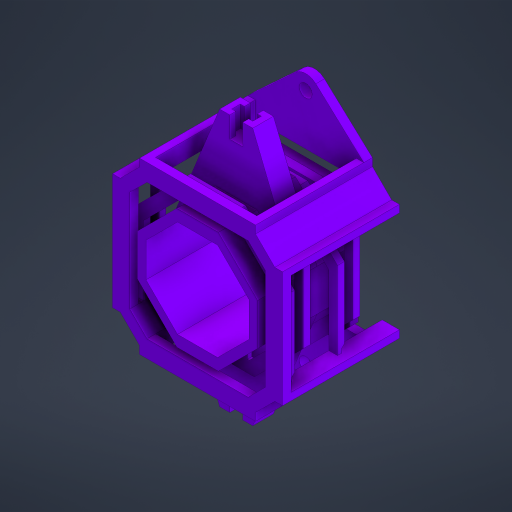
# Autodesk Inventor part: Z Axis Sample V1
Saved by Autodesk Inventor 2023.4 (Build 274418000, 418)
## iProperties
Created: 2022-08-08
Part Number: Z Axis Sample V1
Material: Generic
Document SubType Name: Modeling
Designer: xSibe
Density: 1 g/cm^3
Appearance: Plastic Purple
Author: xSibe
Autodesk Inventor part; units mm, degrees
ref_plane "YZ Plane" through (0, 0, 0) normal (1, 0, 0) x (0, 1, 0)
ref_plane "XZ Plane" through (0, 0, 0) normal (0, 1, 0) x (-1, 0, 0)
ref_plane "XY Plane" through (0, 0, 0) normal (0, 0, 1) x (1, 0, 0)
sketch "Sketch1" plane through (0, 0, 0) normal (0, 0, 1) x (1, 0, 0)
  circle A0 centre (-10, 20.9) radius 1.875 projected
  circle A1 centre (-10, -20.9) radius 1.875 projected
  circle A2 centre (10, 20.9) radius 1.875 projected
  circle A3 centre (10, -20.9) radius 1.875 projected
  circle A4 centre (20.8, -14.4) radius 2.075 projected
  circle A5 centre (20.8, 14.4) radius 2.075 projected
  circle A6 centre (-20.8, 14.4) radius 2.075 projected
  circle A7 centre (-20.8, -14.4) radius 2.075 projected
  line L0 (16.9, -16.9) -> (-16.9, -16.9) projected
  line L1 (-16.9, -16.9) -> (-16.9, 16.9) projected
  line L2 (-16.9, 16.9) -> (16.9, 16.9) projected
  line L3 (16.9, 16.9) -> (16.9, -16.9) projected
  line L4 (-17.05, 24.9) -> (-17.05, 22.55) projected
  line L5 (-17.05, 22.55) -> (-22.55, 17.05) projected
  line L6 (-22.55, 17.05) -> (-24.9, 17.05) projected
  line L7 (-24.9, 17.05) -> (-24.9, -17.05) projected
  line L8 (-24.9, -17.05) -> (-22.55, -17.05) projected
  line L9 (-22.55, -17.05) -> (-17.05, -22.55) projected
  line L10 (-17.05, -22.55) -> (-17.05, -24.9) projected
  line L11 (-17.05, -24.9) -> (17.05, -24.9) projected
  line L12 (17.05, -24.9) -> (17.05, -22.55) projected
  line L13 (17.05, -22.55) -> (22.55, -17.05) projected
  line L14 (22.55, -17.05) -> (24.9, -17.05) projected
  line L15 (24.9, -17.05) -> (24.9, 17.05) projected
  line L16 (24.9, 17.05) -> (22.55, 17.05) projected
  line L17 (22.55, 17.05) -> (17.05, 22.55) projected
  line L18 (17.05, 22.55) -> (17.05, 24.9) projected
  line L19 (17.05, 24.9) -> (-17.05, 24.9) projected
  line L20 (24.725, 16.875) -> (24.725, -16.875)
  line L21 (24.725, -16.875) -> (22.4775, -16.875)
  line L22 (22.4775, -16.875) -> (16.875, -22.4775)
  line L23 (16.875, -22.4775) -> (16.875, -24.725)
  line L24 (16.875, -24.725) -> (-16.875, -24.725)
  line L25 (-16.875, -24.725) -> (-16.875, -22.4775)
  line L26 (-16.875, -22.4775) -> (-22.4775, -16.875)
  line L27 (-22.4775, -16.875) -> (-24.725, -16.875)
  line L28 (-24.725, -16.875) -> (-24.725, 16.875)
  line L29 (-24.725, 16.875) -> (-22.4775, 16.875)
  line L30 (-22.4775, 16.875) -> (-16.875, 22.4775)
  line L31 (-16.875, 22.4775) -> (-16.875, 24.725)
  line L32 (-16.875, 24.725) -> (16.875, 24.725)
  line L33 (16.875, 24.725) -> (16.875, 22.4775)
  line L34 (16.875, 22.4775) -> (22.4775, 16.875)
  line L35 (22.4775, 16.875) -> (24.725, 16.875)
  circle A8 centre (0, 0) radius 12.5
  line L36 (24.725, -16.875) -> (24.725, -24.725)
  line L37 (24.725, -24.725) -> (16.875, -24.725)
  line L38 (24.725, -24.725) -> (14.725, -24.725)
  line L39 (14.725, -24.725) -> (14.725, -19.725)
  line L40 (19.725, -14.725) -> (24.725, -14.725)
  line L41 (24.725, -14.725) -> (24.725, -24.725)
  line L42 (19.725, -14.725) -> (14.725, -19.725)
  line L43 (24.725, 14.725) -> (19.725, 14.725)
  line L44 (14.725, 19.725) -> (19.725, 14.725)
  line L45 (14.725, 19.725) -> (14.725, 24.725)
  line L46 (14.725, 24.725) -> (24.725, 24.725)
  line L47 (24.725, 24.725) -> (24.725, 14.725)
  line L48 (-14.725, 24.725) -> (-14.725, 19.725)
  line L49 (-19.725, 14.725) -> (-14.725, 19.725)
  line L50 (-19.725, 14.725) -> (-24.725, 14.725)
  line L51 (-24.725, 14.725) -> (-24.725, 24.725)
  line L52 (-24.725, 24.725) -> (-14.725, 24.725)
  line L53 (-24.725, -14.725) -> (-19.725, -14.725)
  line L54 (-14.725, -19.725) -> (-19.725, -14.725)
  line L55 (-14.725, -19.725) -> (-14.725, -24.725)
  line L56 (-14.725, -24.725) -> (-24.725, -24.725)
  line L57 (-24.725, -24.725) -> (-24.725, -14.725)
  line L58 (14.725, -19.725) -> (-14.725, -19.725)
  line L59 (-14.725, -19.725) -> (-14.725, -24.725)
  line L60 (-14.725, -24.725) -> (14.725, -24.725)
  line L61 (14.725, -24.725) -> (14.725, -19.725)
  line L62 (-19.725, -14.725) -> (-24.725, -14.725)
  line L63 (-24.725, -14.725) -> (-24.725, 14.725)
  line L64 (-24.725, 14.725) -> (-19.725, 14.725)
  line L65 (-19.725, 14.725) -> (-19.725, -14.725)
  line L66 (-14.725, 19.725) -> (14.725, 19.725)
  line L67 (14.725, 19.725) -> (14.725, 24.725)
  line L68 (14.725, 24.725) -> (-14.725, 24.725)
  line L69 (-14.725, 24.725) -> (-14.725, 19.725)
  line L70 (19.725, 14.725) -> (24.725, 14.725)
  line L71 (24.725, 14.725) -> (24.725, -14.725)
  line L72 (24.725, -14.725) -> (19.725, -14.725)
  line L73 (19.725, -14.725) -> (19.725, 14.725)
  point P0 (16.875, -16.875)
  point P1 (14.725, -14.725)
  dimension "d0" = 0.175
  dimension "d3" = 25
  dimension "d24" = 10
  dimension "d25" = 10
  dimension "d26" = 5
  dimension "d27" = 5
  dimension "d30" = 360
  constraints: 108 end point, 10 parallel, 6 perpendicular, 5 horizontal, 2 point on line, 1 centre point, 1 coincident, 1 vertical, 56 other
  measures "d0" distance between parallel lines of L15 L20
  measures "d3" diameter of A8
  measures "d24" distance of point (14.725, -14.725) L40.end
  measures "d25" distance of L38.end point (14.725, -14.725)
  measures "d26" distance of L40.start point (14.725, -14.725)
  measures "d27" distance of L39.end point (14.725, -14.725)
ref_plane "Work Plane1" through (-24.9, -24.9, 7.7) normal (0, 0, 1) x (1, 0, 0)
extrude "Extrusion1" add sketch "Sketch1" along normal blind 2.5 from surface at 7.7 contours A0 L66 | A0 L66 L48 L32 L45 A2 | L49 A6 L50 L28 L29 L30 L31 L32 L48 | A2 L66 | L49 L50 A6 | L32 L33 L34 L35 L20 L43 A5 L44 L45 | L50 L65 A6 | A6 L65 A7 L53 L28 L50 | A5 L43 L44 | L65 L53 A7 | L53 A7 L54 L55 L24 L25 L26 L27 L28 | L43 L20 L40 A4 L73 A5 | A5 L73 L43 | L53 L54 A7 | A4 L40 L73 | L20 L21 L22 L23 L24 L39 L42 A4 L40 | L42 L40 A4 | L58 A1 A3 L39 L24 L55 | L58 A1 | A3 L58 picked at (-10.1758, 21.5261) picked at (10.0076, 20.8619) picked at (-9.9136, -20.7357) picked at (10.3659, -21.7168)
sketch "Sketch2" plane through (0, 0, 0) normal (0, 0, 1) x (1, 0, 0)
  line L0 (22.4775, 16.875) -> (24.725, 16.875) projected
  line L1 (16.875, 22.4775) -> (22.4775, 16.875) projected
  line L2 (16.875, 24.725) -> (16.875, 22.4775) projected
  line L3 (-16.875, 24.725) -> (16.875, 24.725) projected
  line L4 (-16.875, 22.4775) -> (-16.875, 24.725) projected
  line L5 (-22.4775, 16.875) -> (-16.875, 22.4775) projected
  line L6 (-24.725, 16.875) -> (-22.4775, 16.875) projected
  line L7 (-24.725, -16.875) -> (-24.725, 16.875) projected
  line L8 (-22.4775, -16.875) -> (-24.725, -16.875) projected
  line L9 (-16.875, -22.4775) -> (-22.4775, -16.875) projected
  line L10 (-16.875, -24.725) -> (-16.875, -22.4775) projected
  line L11 (16.875, -24.725) -> (-16.875, -24.725) projected
  line L12 (16.875, -22.4775) -> (16.875, -24.725) projected
  line L13 (22.4775, -16.875) -> (16.875, -22.4775) projected
  line L14 (24.725, -16.875) -> (22.4775, -16.875) projected
  line L15 (24.725, 16.875) -> (24.725, -16.875) projected
  line L16 (-16.875, -24.725) -> (-24.725, -24.725)
  line L17 (-24.725, -24.725) -> (-24.725, -16.875)
  line L18 (-24.725, -24.725) -> (-14.725, -24.725)
  line L19 (-14.725, -24.725) -> (-14.725, -19.725)
  line L20 (-19.725, -14.725) -> (-24.725, -14.725)
  line L21 (-24.725, -14.725) -> (-24.725, -24.725)
  line L22 (-14.725, -19.725) -> (-19.725, -14.725)
  line L23 (24.725, -14.725) -> (19.725, -14.725)
  line L24 (19.725, -14.725) -> (14.725, -19.725)
  line L25 (14.725, -19.725) -> (14.725, -24.725)
  line L26 (24.725, -24.725) -> (16.875, -24.725)
  line L27 (24.725, -24.725) -> (24.725, -14.725)
  line L28 (14.725, 24.725) -> (14.725, 19.725)
  line L29 (14.725, 19.725) -> (19.725, 14.725)
  line L30 (19.725, 14.725) -> (24.725, 14.725)
  line L31 (24.725, 24.725) -> (24.725, 16.875)
  line L32 (24.725, 24.725) -> (14.725, 24.725)
  line L33 (-24.725, 14.725) -> (-19.725, 14.725)
  line L34 (-19.725, 14.725) -> (-14.725, 19.725)
  line L35 (-14.725, 19.725) -> (-14.725, 24.725)
  line L36 (-24.725, 24.725) -> (-16.875, 24.725)
  line L37 (-24.725, 24.725) -> (-24.725, 14.725)
  line L38 (24.725, 14.725) -> (19.725, 14.725)
  line L39 (19.725, 14.725) -> (19.725, -14.725)
  line L40 (19.725, -14.725) -> (24.725, -14.725)
  line L41 (24.725, -14.725) -> (24.725, 14.725)
  line L42 (14.725, -19.725) -> (-14.725, -19.725)
  line L43 (-14.725, -19.725) -> (-14.725, -24.725)
  line L44 (-14.725, -24.725) -> (14.725, -24.725)
  line L45 (14.725, -24.725) -> (14.725, -19.725)
  line L46 (-19.725, -14.725) -> (-24.725, -14.725)
  line L47 (-24.725, -14.725) -> (-24.725, 14.725)
  line L48 (-24.725, 14.725) -> (-19.725, 14.725)
  line L49 (-19.725, 14.725) -> (-19.725, -14.725)
  line L50 (-14.725, 19.725) -> (14.725, 19.725)
  line L51 (14.725, 19.725) -> (14.725, 24.725)
  line L52 (14.725, 24.725) -> (-14.725, 24.725)
  line L53 (-14.725, 24.725) -> (-14.725, 19.725)
  point P0 (0, 0)
  point P1 (-14.725, -14.725)
  dimension "d12" = 10
  dimension "d13" = 10
  dimension "d14" = 5
  dimension "d15" = 5
  dimension "d18" = 360
  constraints: 76 end point, 10 parallel, 6 horizontal, 6 perpendicular, 2 point on line, 45 other
  measures "d12" distance of L20.end point (-14.725, -14.725)
  measures "d13" distance of point (-14.725, -14.725) L18.end
  measures "d14" distance of L19.end point (-14.725, -14.725)
  measures "d15" distance of L20.start point (-14.725, -14.725)
extrude "Extrusion2" add sketch "Sketch2" along normal blind 31.5 from surface at 10.2 contours L0 L15 L30 L29 L28 L3 L2 L1 | L15 L14 L13 L12 L11 L25 L24 L23 | L35 L34 L33 L7 L6 L5 L4 L3 | L19 L11 L10 L9 L8 L7 L20 L22
extrude "Extrusion3" add sketch "Sketch2" against normal blind 2.5 from surface at 41.7 contours L15 L23 L39 L30 | L28 L50 L35 L3 | L25 L11 L19 L42 | L49 L20 L7 L33
sketch "Sketch3" plane through (0, 0, 0) normal (0, 0, 1) x (1, 0, 0)
  line L0 (-14.725, 19.725) -> (-19.725, 14.725) projected
  line L1 (14.725, 19.725) -> (-14.725, 19.725) projected
  line L2 (19.725, 14.725) -> (14.725, 19.725) projected
  line L3 (14.725, -19.725) -> (19.725, -14.725) projected
  line L4 (-14.725, -19.725) -> (14.725, -19.725) projected
  line L5 (-19.725, -14.725) -> (-14.725, -19.725) projected
  line L6 (-24.725, -16.875) -> (-24.725, 16.875) projected
  line L7 (-22.4775, -16.875) -> (-24.725, -16.875) projected
  line L8 (-16.875, -22.4775) -> (-22.4775, -16.875) projected
  line L9 (-16.875, -24.725) -> (-16.875, -22.4775) projected
  line L10 (16.875, -24.725) -> (-16.875, -24.725) projected
  line L11 (16.875, -22.4775) -> (16.875, -24.725) projected
  line L12 (22.4775, -16.875) -> (16.875, -22.4775) projected
  line L13 (24.725, -16.875) -> (22.4775, -16.875) projected
  line L14 (24.725, 16.875) -> (24.725, -16.875) projected
  line L15 (22.4775, 16.875) -> (24.725, 16.875) projected
  line L16 (16.875, 22.4775) -> (22.4775, 16.875) projected
  line L17 (16.875, 24.725) -> (16.875, 22.4775) projected
  line L18 (-16.875, 24.725) -> (16.875, 24.725) projected
  line L19 (-16.875, 22.4775) -> (-16.875, 24.725) projected
  line L20 (-22.4775, 16.875) -> (-16.875, 22.4775) projected
  line L21 (-24.725, 16.875) -> (-22.4775, 16.875) projected
  circle A0 centre (0, 0) radius 13.25
  circle A1 centre (0, 0) radius 18.25
  line L22 (13.25, 18.25) -> (-13.25, 18.25)
  line L23 (-18.25, 13.25) -> (-18.25, -13.25)
  line L24 (-13.25, -18.25) -> (13.25, -18.25)
  line L25 (18.25, -13.25) -> (18.25, 13.25)
  line L26 (18.25, 18.25) -> (-18.25, -18.25) construction
  line L27 (-18.25, 18.25) -> (18.25, -18.25) construction
  line L28 (-14.725, -19.725) -> (-14.725, -24.725) projected
  line L29 (14.725, -24.725) -> (-14.725, -24.725) projected
  line L30 (14.725, -24.725) -> (14.725, -19.725) projected
  line L31 (-14.725, -19.725) -> (14.725, -19.725) projected
  line L32 (24.725, 14.725) -> (19.725, 14.725) projected
  line L33 (19.725, -14.725) -> (19.725, 14.725) projected
  line L34 (19.725, -14.725) -> (24.725, -14.725) projected
  line L35 (24.725, 14.725) -> (24.725, -14.725) projected
  line L36 (-19.725, 14.725) -> (-24.725, 14.725) projected
  line L37 (-24.725, -14.725) -> (-24.725, 14.725) projected
  line L38 (-24.725, -14.725) -> (-19.725, -14.725) projected
  line L39 (-19.725, 14.725) -> (-19.725, -14.725) projected
  line L40 (-14.725, 24.725) -> (-14.725, 19.725) projected
  line L41 (14.725, 19.725) -> (-14.725, 19.725) projected
  line L42 (14.725, 19.725) -> (14.725, 24.725) projected
  line L43 (-14.725, 24.725) -> (14.725, 24.725) projected
  line L44 (18.25, -13.25) -> (13.25, -18.25)
  line L45 (-13.25, -18.25) -> (-18.25, -13.25)
  line L46 (-18.25, 13.25) -> (-13.25, 18.25)
  line L47 (13.25, 18.25) -> (18.25, 13.25)
  line L48 (10, 14.1625) -> (-10, 14.1625)
  line L49 (-10, 14.1625) -> (-10, -14.1625)
  line L50 (-10, -14.1625) -> (10, -14.1625)
  line L51 (10, -14.1625) -> (10, 14.1625)
  line L52 (10, 14.1625) -> (-10, -14.1625) construction
  line L53 (-10, 14.1625) -> (10, -14.1625) construction
  line L54 (5, 15) -> (-5, 15)
  line L55 (-15, 5) -> (-15, -5)
  line L56 (-5, -15) -> (5, -15)
  line L57 (15, -5) -> (15, 5)
  line L58 (15, 15) -> (-15, -15) construction
  line L59 (-15, 15) -> (15, -15) construction
  line L60 (15, -5) -> (5, -15)
  line L61 (-5, -15) -> (-15, -5)
  line L62 (-15, 5) -> (-5, 15)
  line L63 (5, 15) -> (15, 5)
  line L64 (6.0355, -17.5) -> (17.5, -6.0355)
  line L65 (17.5, -6.0355) -> (17.5, 6.0355)
  line L66 (17.5, 6.0355) -> (6.0355, 17.5)
  line L67 (6.0355, 17.5) -> (-6.0355, 17.5)
  line L68 (-6.0355, 17.5) -> (-17.5, 6.0355)
  line L69 (-17.5, 6.0355) -> (-17.5, -6.0355)
  line L70 (-17.5, -6.0355) -> (-6.0355, -17.5)
  line L71 (-6.0355, -17.5) -> (6.0355, -17.5)
  line L72 (6.0355, 17.5) -> (14, 17.5)
  line L73 (-6.0355, 17.5) -> (-14, 17.5)
  line L74 (10, 15.6625) -> (-10, 15.6625)
  line L75 (-10, 15.6625) -> (-10, 12.6625)
  line L76 (-10, 12.6625) -> (10, 12.6625)
  line L77 (10, 12.6625) -> (10, 15.6625)
  line L78 (10, 15.6625) -> (-10, 12.6625) construction
  line L79 (-10, 15.6625) -> (10, 12.6625) construction
  line L80 (10, -12.6625) -> (-10, -12.6625)
  line L81 (-10, -12.6625) -> (-10, -15.6625)
  line L82 (-10, -15.6625) -> (10, -15.6625)
  line L83 (10, -15.6625) -> (10, -12.6625)
  line L84 (10, -12.6625) -> (-10, -15.6625) construction
  line L85 (-10, -12.6625) -> (10, -15.6625) construction
  circle A2 centre (0, 0) radius 12.6625
  line L86 (-19.725, 14.725) -> (-19.725, -14.725) projected
  line L87 (19.725, -14.725) -> (19.725, 14.725) projected
  point P0 (-18.25, 10)
  point P1 (-18.25, -10)
  point P2 (18.25, -10)
  point P3 (18.25, 10)
  point P4 (15, 10.3953)
  point P5 (10.3953, 15)
  point P6 (-15, 10.3953)
  point P7 (-10.3953, 15)
  point P8 (-10.3953, -15)
  point P9 (-15, -10.3953)
  point P10 (15, -10.3953)
  point P11 (10.3953, -15)
  point P12 (10, 10)
  point P13 (10, -10)
  point P14 (-10, -10)
  point P15 (-10, 10)
  point P16 (-5.8375, -14.1625)
  point P17 (-5.8375, 14.1625)
  point P18 (5.8375, 14.1625)
  point P19 (5.8375, -14.1625)
  point P20 (0, 14.1625)
  point P21 (0, -14.1625)
  point P22 (-10, 12.6625)
  point P23 (10, 12.6625)
  point P24 (10, 14.1625)
  dimension "d32" = 26.5
  dimension "d33" = 5
  dimension "d36" = 5
  dimension "d37" = 5
  dimension "d38" = 5
  dimension "d39" = 5
  dimension "d40" = 5
  dimension "d41" = 5
  dimension "d42" = 5
  dimension "d43" = 5
  dimension "d49" = 20
  dimension "d50" = 28.325
  dimension "d57" = 30
  dimension "d58" = 30
  dimension "d59" = 10
  dimension "d60" = 10
  dimension "d61" = 10
  dimension "d62" = 10
  dimension "d63" = 10
  dimension "d64" = 10
  dimension "d65" = 10
  dimension "d66" = 10
  dimension "d67" = 2.5
  dimension "d120" = 20
  dimension "d121" = 3
  dimension "d122" = 20
  dimension "d123" = 3
  constraints: 96 end point, 19 point on line, 12 midpoint, 12 parallel, 7 perpendicular, 5 horizontal, 3 centre point, 3 tangent, 2 coincident, 7 other
  measures "d32" diameter of A0
  measures "d33" radial gap between concentric circles of A0 A1
  measures "d36" distance of L25.start L27.end
  measures "d37" distance of L24.end L27.end
  measures "d38" distance of L24.start L26.end
  measures "d39" distance of L23.end L26.end
  measures "d40" distance of L23.start L27.start
  measures "d41" distance of L22.end L27.start
  measures "d42" distance of L22.start L26.start
  measures "d43" distance of L25.end L26.start
  measures "d49" distance of L50.end L49.end
  measures "d50" distance of L49.end L48.end
  measures "d57" distance of L59.end L58.end
  measures "d58" distance of L58.end L59.start
  measures "d59" distance of L57.start L59.end
  measures "d60" distance of L56.end L59.end
  measures "d61" distance of L56.start L58.end
  measures "d62" distance of L55.end L58.end
  measures "d63" distance of L55.start L59.start
  measures "d64" distance of L54.end L59.start
  measures "d65" distance of L54.start L58.start
  measures "d66" distance of L57.end L58.start
  measures "d67" distance between parallel lines of L56 L71
  measures "d120" distance of L76.end L75.end
  measures "d121" distance of L75.end L74.end
  measures "d122" distance of L82.end L81.end
  measures "d123" distance of L81.end L80.end
ref_plane "Work Plane2" through (16.875, 24.725, 14.45) normal (0, 0, -1) x (-1, 0, 0)
extrude "Extrusion4" add sketch "Sketch3" along normal mid plane 2.5 from surface at 14.45 contours A0 L51 A2 | A0 L51 L63 L57 L60 | L51 A2 L76 A0 | A0 L76 L63 L51 | L51 L60 L80 A0 | A0 L80 A2 L51 | L76 A0 | A0 L76 L62 L48 L63 | L63 L76 L51 | L51 L66 A1 L65 L64 L60 L57 L63 | L80 L60 L50 L61 A0 | A0 L80 | L51 L80 L60 | L76 A2 L49 A0 | A0 L49 L62 L76 | L63 L48 L66 L51 L76 | L80 L61 L49 A0 | A0 L49 A2 L80 | L80 L51 L64 L50 L60 | L49 A2 A0 | A0 L49 L61 L55 L62 | L76 L49 L68 L48 L62 | L62 L49 L76 | L63 L54 L62 L48 L68 L74 L66 | L48 L62 L54 L63 | L66 L48 L51 | L51 L77 A1 L66 | L80 L49 L61 | L61 L50 L70 L49 L80 | L60 L56 L61 L50 | L50 L64 L82 L70 L61 L56 L60 | L64 A1 L83 L51 | L51 L50 L64 | L62 L55 L61 L49 L70 A1 L69 L68 | L66 L74 A1 L77 L48 | L66 L65 A1 | A1 L77 L74 L66 L72 L47 L25 L65 | L50 L83 A1 L82 L64 | L64 L65 A1 L25 L44 L24 L71 L82 L83 | A1 L65 L64 | L68 L49 L48 | L48 L75 A1 L74 L68 | L68 A1 L75 L49 | L74 L68 A1 L67 L66 | L66 A1 L74 | A1 L74 L77 | A1 L65 | L70 L82 A1 L81 L50 | L50 L49 L70 | L49 L81 A1 L70 | L82 A1 L64 | L64 A1 L71 L70 L82 | L83 L82 A1 | L74 A1 L68 | L68 L69 A1 L23 L46 L73 L74 L75 | A1 L69 L68 | A1 L67 L66 | L70 A1 L82 | L70 L69 A1 | A1 L81 L82 L70 L71 L24 L45 L23 L69 | L64 L71 A1 | L75 L74 A1 | L68 L67 A1 | L69 A1 | L67 A1 | A1 L22 L47 L72 L67 | A1 L82 L81 | A1 L71 L70 | A1 L71 | L67 L73 L46 L22 A1
extrude "Extrusion5" add sketch "Sketch3" along normal up to surface (26 mm away) from surface at 15.7 contours L63 L76 L51 | L51 L66 A1 L65 L64 L60 L57 L63 | L51 L80 L60 | L63 L48 L66 L51 L76 | L80 L51 L64 L50 L60 | L76 L49 L68 L48 L62 | L62 L49 L76 | L63 L54 L62 L48 L68 L74 L66 | L48 L62 L54 L63 | L80 L49 L61 | L61 L50 L70 L49 L80 | L60 L56 L61 L50 | L50 L64 L82 L70 L61 L56 L60 | L62 L55 L61 L49 L70 A1 L69 L68 | L66 L65 A1 | A1 L65 L64 | L74 L68 A1 L67 L66 | L64 A1 L71 L70 L82 | A1 L69 L68 | A1 L67 L66 | L70 L69 A1 | L64 L71 A1 | L68 L67 A1 | A1 L71 L70
extrude "Extrusion6" add sketch "Sketch3" against normal blind 5 from surface at 13.2 contours L76 A0 | A0 L76 L62 L48 L63 | L80 L60 L50 L61 A0 | A0 L80 | L63 L48 L66 L51 L76 | L80 L51 L64 L50 L60 | L76 L49 L68 L48 L62 | L63 L54 L62 L48 L68 L74 L66 | L48 L62 L54 L63 | L66 L48 L51 | L61 L50 L70 L49 L80 | L60 L56 L61 L50 | L50 L64 L82 L70 L61 L56 L60 | L51 L50 L64 | L66 L74 A1 L77 L48 | L50 L83 A1 L82 L64 | L68 L49 L48 | L48 L75 A1 L74 L68 | A1 L74 L77 | L70 L82 A1 L81 L50 | L50 L49 L70 | L83 L82 A1 | L75 L74 A1 | A1 L82 L81
sketch "Sketch4" plane through (0, 0, 0) normal (0, 0, 1) x (1, 0, 0)
  line L0 (-14.725, 24.725) -> (-14.725, 19.725) projected
  line L1 (14.725, 19.725) -> (-14.725, 19.725) projected
  line L2 (14.725, 19.725) -> (14.725, 24.725) projected
  line L3 (-14.725, 24.725) -> (14.725, 24.725) projected
  line L4 (24.725, 14.725) -> (19.725, 14.725) projected
  line L5 (19.725, -14.725) -> (19.725, 14.725) projected
  line L6 (19.725, -14.725) -> (24.725, -14.725) projected
  line L7 (24.725, 14.725) -> (24.725, -14.725) projected
  line L8 (-14.725, -19.725) -> (-14.725, -24.725) projected
  line L9 (14.725, -24.725) -> (-14.725, -24.725) projected
  line L10 (14.725, -24.725) -> (14.725, -19.725) projected
  line L11 (-14.725, -19.725) -> (14.725, -19.725) projected
  line L12 (-19.725, 14.725) -> (-24.725, 14.725) projected
  line L13 (-24.725, -14.725) -> (-24.725, 14.725) projected
  line L14 (-24.725, -14.725) -> (-19.725, -14.725) projected
  line L15 (-19.725, 14.725) -> (-19.725, -14.725) projected
  arc A0 (-4.0214, 12.625) -> (-4.0214, -12.625) centre (0, 0) ccw projected
  line L16 (-15, -5) -> (-5.8375, -14.1625) projected
  line L17 (-5.8375, 14.1625) -> (-15, 5) projected
  line L18 (5.8375, 14.1625) -> (-5.8375, 14.1625) projected
  line L19 (15, 5) -> (5.8375, 14.1625) projected
  line L20 (5.8375, -14.1625) -> (15, -5) projected
  line L21 (-5.8375, -14.1625) -> (5.8375, -14.1625) projected
  line L22 (-6.0355, -17.5) -> (-17.5, -6.0355) projected
  line L23 (6.0355, -17.5) -> (-6.0355, -17.5) projected
  line L24 (17.5, -6.0355) -> (6.0355, -17.5) projected
  line L25 (17.5, 6.0355) -> (17.5, -6.0355) projected
  line L26 (6.0355, 17.5) -> (17.5, 6.0355) projected
  line L27 (-6.0355, 17.5) -> (6.0355, 17.5) projected
  line L28 (-17.5, 6.0355) -> (-6.0355, 17.5) projected
  line L29 (-17.5, -6.0355) -> (-17.5, 6.0355) projected
  line L30 (6.0355, -17.5) -> (-6.0355, -17.5)
  line L31 (-6.0355, -17.5) -> (-6.0355, -18.75)
  line L32 (-6.0355, -18.75) -> (6.0355, -18.75)
  line L33 (6.0355, -18.75) -> (6.0355, -17.5)
  line L34 (-7.33, -20.625) -> (-20.625, -7.33)
  line L35 (-20.625, -7.33) -> (-20.625, 7.33)
  line L36 (-20.625, 7.33) -> (-7.33, 20.625)
  line L37 (-7.33, 20.625) -> (7.33, 20.625)
  line L38 (7.33, 20.625) -> (20.625, 7.33)
  line L39 (20.625, 7.33) -> (20.625, -7.33)
  line L40 (20.625, -7.33) -> (7.33, -20.625)
  line L41 (7.33, -20.625) -> (-7.33, -20.625)
  line L42 (-6.5533, -18.75) -> (-18.75, -6.5533)
  line L43 (-18.75, -6.5533) -> (-18.75, 6.5533)
  line L44 (-18.75, 6.5533) -> (-6.5533, 18.75)
  line L45 (-6.5533, 18.75) -> (6.5533, 18.75)
  line L46 (6.5533, 18.75) -> (18.75, 6.5533)
  line L47 (18.75, 6.5533) -> (18.75, -6.5533)
  line L48 (18.75, -6.5533) -> (6.5533, -18.75)
  line L49 (6.5533, -18.75) -> (-6.5533, -18.75)
  line L50 (18.75, -6.5533) -> (20.625, -4.6783)
  line L51 (0, -18.75) -> (0, -17.5)
  line L52 (22.225, -7.9927) -> (22.225, 7.9927)
  line L53 (22.225, 7.9927) -> (7.9927, 22.225)
  line L54 (7.9927, 22.225) -> (-7.9927, 22.225)
  line L55 (-7.9927, 22.225) -> (-22.225, 7.9927)
  line L56 (-22.225, 7.9927) -> (-22.225, -7.9927)
  line L57 (-22.225, -7.9927) -> (-7.9927, -22.225)
  line L58 (-7.9927, -22.225) -> (7.9927, -22.225)
  line L59 (7.9927, -22.225) -> (22.225, -7.9927)
  line L60 (22.225, 7.9927) -> (22.225, 14.725)
  line L61 (-18.75, -6.5533) -> (-20.625, -4.6783)
  line L62 (-22.225, 7.9927) -> (-22.225, 14.725)
  line L63 (22.225, 14.725) -> (19.725, 14.725)
  line L64 (19.725, 14.725) -> (19.725, 13.475)
  line L65 (19.725, 13.475) -> (22.225, 13.475)
  line L66 (22.225, 13.475) -> (22.225, 14.725)
  line L67 (-22.225, 14.725) -> (-19.725, 14.725)
  line L68 (-19.725, 14.725) -> (-19.725, 13.475)
  line L69 (-19.725, 13.475) -> (-22.225, 13.475)
  line L70 (-22.225, 13.475) -> (-22.225, 14.725)
  line L71 (-15, 5) -> (-15, -5) projected
  line L72 (15, -5) -> (15, 5) projected
  point P0 (-19.725, 8.23)
  point P1 (19.725, -5.5783)
  point P2 (-19.725, -5.5783)
  point P3 (-19.725, 14.725)
  point P4 (6.0354, -18.75)
  point P5 (-10, -8.6927)
  point P6 (10, -8.6927)
  point P7 (10, 8.6927)
  dimension "d71" = 1.25
  dimension "d72" = 3.125
  dimension "d73" = 1.25
  dimension "d74" = 1.6
  dimension "d78" = 1.25
  constraints: 82 end point, 6 symmetric about line, 4 parallel, 3 midpoint, 2 horizontal, 2 perpendicular, 2 point on line, 1 collinear, 21 other
  measures "d71" distance of L22.start L31.end
  measures "d72" distance between parallel lines of L23 L41
  measures "d73" distance between parallel lines of L23 L49
  measures "d74" distance between parallel lines of L39 L52
  measures "d78" distance of L64.end L63.end
ref_plane "Work Plane3" through (-13.25, -18.25, 18.7) normal (0, 0, 1) x (1, 0, 0)
extrude "Extrusion7" add sketch "Sketch4" against normal blind 2 from surface at 18.7 contours L55 L62 L69 L15 | L15 L36 L35 L34 L57 L56 L55 | L15 L61 L35 L36 | L53 L52 L59 L5 L40 L39 L38 | L5 L65 L60 L53 | L38 L39 L50 L5 | L61 L42 L49 L32 L48 L50 L5 L40 L11 L34 L15 | L15 L34 L35 L61 | L50 L39 L40 L5 | L34 L11 L57 L15 | L5 L59 L11 L40 | L34 L41 L40 L11 L59 L58 L57 | L11 L40 L41 L34
extrude "Extrusion8" add sketch "Sketch4" against normal blind 1.25 from surface at 18.7 contours L69 L62 L12 L15 | L5 L4 L60 L65 | L31 L23 L51 L32 | L32 L51 L23 L33
sketch "Sketch5" plane through (0, 0, 0) normal (0, 0, 1) x (1, 0, 0)
  line L0 (6.0355, -18.75) -> (6.5533, -18.75) projected
  line L1 (22.225, 14.725) -> (22.225, -7.9927) projected
  line L2 (7.9927, -22.225) -> (-7.9927, -22.225) projected
  line L3 (-22.225, -7.9927) -> (-22.225, 14.725) projected
  line L4 (22.225, 14.725) -> (22.225, 13.475) projected
  line L5 (19.725, 14.725) -> (22.225, 14.725) projected
  line L6 (19.725, 13.475) -> (19.725, 14.725) projected
  line L7 (-19.725, 14.725) -> (-19.725, 13.475) projected
  line L8 (-22.225, 14.725) -> (-19.725, 14.725) projected
  line L9 (-22.225, 13.475) -> (-22.225, 14.725) projected
  line L10 (-6.0355, -18.75) -> (-6.0355, -17.5) projected
  line L11 (6.0355, -17.5) -> (6.0355, -18.75) projected
  line L12 (0, 0) -> (-19.725, 0)
  line L13 (-19.725, -14.725) -> (-19.725, 5.5783)
  line L14 (-19.725, 5.5783) -> (-6.5533, 18.75)
  line L15 (-6.5533, 18.75) -> (-6.0355, 18.75)
  line L16 (-6.0355, 18.75) -> (-6.0355, 17.5)
  line L17 (-6.0355, 17.5) -> (6.0355, 17.5)
  line L18 (6.0355, 17.5) -> (6.0355, 18.75)
  line L19 (6.0355, 18.75) -> (6.5533, 18.75)
  line L20 (6.5533, 18.75) -> (19.725, 5.5783)
  line L21 (19.725, 5.5783) -> (19.725, -14.725)
  line L22 (19.725, -14.725) -> (22.225, -14.725)
  line L23 (22.225, -14.725) -> (22.225, 7.9927)
  line L24 (22.225, 7.9927) -> (7.9927, 22.225)
  line L25 (7.9927, 22.225) -> (-7.9927, 22.225)
  line L26 (-7.9927, 22.225) -> (-22.225, 7.9927)
  line L27 (-22.225, 7.9927) -> (-22.225, -14.725)
  line L28 (-22.225, -14.725) -> (-19.725, -14.725)
  line L29 (22.225, -14.725) -> (22.225, -13.475)
  line L30 (19.725, -14.725) -> (22.225, -14.725)
  line L31 (19.725, -13.475) -> (19.725, -14.725)
  line L32 (22.225, -13.475) -> (19.725, -13.475)
  line L33 (-19.725, -14.725) -> (-19.725, -13.475)
  line L34 (-22.225, -14.725) -> (-19.725, -14.725)
  line L35 (-22.225, -13.475) -> (-22.225, -14.725)
  line L36 (-19.725, -13.475) -> (-22.225, -13.475)
  line L37 (-6.0355, 18.75) -> (-6.0355, 17.5)
  line L38 (6.0355, 18.75) -> (-6.0355, 18.75)
  line L39 (6.0355, 17.5) -> (6.0355, 18.75)
  line L40 (-6.0355, 17.5) -> (6.0355, 17.5)
  line L41 (-6.0355, -17.5) -> (6.0355, -17.5) projected
  line L42 (22.225, -7.9927) -> (7.9927, -22.225) projected
  line L43 (-19.725, -5.5783) -> (-6.5533, -18.75) projected
  line L44 (6.5533, -18.75) -> (19.725, -5.5783) projected
  line L45 (-7.9927, -22.225) -> (-22.225, -7.9927) projected
  line L46 (6.0355, -18.75) -> (-6.0355, -18.75) projected
  line L47 (-19.725, 13.475) -> (-22.225, 13.475) projected
  line L48 (22.225, 13.475) -> (19.725, 13.475) projected
  line L49 (-22.225, 14.725) -> (-19.725, 14.725) projected
  line L50 (-6.0355, -18.75) -> (-6.0355, -17.5) projected
  line L51 (-6.0355, -17.5) -> (6.0355, -17.5) projected
  line L52 (6.0355, -17.5) -> (6.0355, -18.75) projected
  line L53 (19.725, 14.725) -> (22.225, 14.725) projected
  line L54 (-6.5533, -18.75) -> (-6.0355, -18.75) projected
  line L55 (-19.725, 14.725) -> (-19.725, -5.5783) projected
  line L56 (19.725, -5.5783) -> (19.725, 14.725) projected
  point P0 (22.225, -0.226)
  point P1 (-22.225, -0.0977)
  point P2 (19.725, -10.4927)
  point P3 (-19.725, -10.4927)
  point P4 (-22.225, 0)
  point P5 (22.225, 0.0001)
  point P6 (19.725, 10.4927)
  point P7 (19.725, 5.5783)
  point P8 (-19.725, 10.4927)
  point P9 (-19.725, 5.5783)
  point P10 (-19.725, -5.5783)
  constraints: 58 end point, 18 symmetric about line
ref_plane "Work Plane4" through (-13.25, -18.25, 23.2) normal (0, 0, 1) x (1, 0, 0)
extrude "Extrusion9" add sketch "Sketch5" against normal blind 2 from surface at 23.2 contours L21 L56 L24 L1 L42 | L20 L19 L38 L15 L14 L55 L26 L25 L24 L56 | L42 L23 L32 L21 | L13 L45 L3 L26 L55 | L13 L36 L27 L45
extrude "Extrusion10" add sketch "Sketch5" against normal blind 1.25 from surface at 23.2 contours L32 L23 L22 L21 | L18 L17 L16 L38 | L13 L28 L27 L36
chamfer "Chamfer3" distance 0.75 angle 45 10 edges at (20.975, -13.475, 21.2) (20.975, 13.475, 16.7) (6.2944, 18.75, 21.2) (0, 18.75, 21.2) (-6.2944, 18.75, 21.2) (-20.975, 13.475, 16.7) (-20.975, -13.475, 21.2) (6.2943, -18.75, 16.7) (-6.2944, -18.75, 16.7) (-0.0001, -18.75, 16.7)
pattern_linear "Rectangular Pattern1" count 2 spacing 14.5 along (0, 0, 1) of "Extrusion10", "Extrusion9", "Extrusion8", "Extrusion7", "Chamfer3"
sketch "Sketch6" plane through (0, 0, 0) normal (0, 1, 0) x (-1, 0, 0)
  line L0 (-6.0355, 23.2) -> (-6.0355, 36.45) projected
  line L1 (6.0355, 15.7) -> (-6.0355, 15.7) projected
  line L2 (6.0355, 23.2) -> (6.0355, 36.45) projected
  line L3 (17.5, 15.7) -> (6.0355, 15.7) projected
  line L4 (17.5, 15.7) -> (17.5, 41.7) projected
  line L5 (17.5, 41.7) -> (6.0355, 41.7) projected
  line L6 (-17.5, 15.7) -> (-17.5, 41.7) projected
  line L7 (-6.0355, 15.7) -> (-17.5, 15.7) projected
  line L8 (-6.0355, 21.95) -> (-6.0355, 23.2) projected
  line L9 (-6.0355, 41.7) -> (-17.5, 41.7) projected
  line L10 (-18.25, 13.2) -> (-13.25, 13.2) projected
  line L11 (-18.25, 15.7) -> (-13.25, 15.7) projected
  line L12 (-18.25, 13.2) -> (-18.25, 15.7) projected
  line L13 (13.25, 13.2) -> (18.25, 13.2) projected
  line L14 (18.25, 13.2) -> (18.25, 15.7) projected
  line L15 (13.25, 15.7) -> (18.25, 15.7) projected
  line L16 (0, 26.95) -> (0, 27.95)
  line L17 (-3.0625, 26.2) -> (3.0625, 26.2)
  line L18 (3.0625, 26.2) -> (3.0625, 28.7)
  line L19 (3.0625, 28.7) -> (-3.0625, 28.7)
  line L20 (-3.0625, 28.7) -> (-3.0625, 26.2)
  line L21 (-3.0625, 26.2) -> (3.0625, 28.7) construction
  line L22 (3.0625, 26.2) -> (-3.0625, 28.7) construction
  line L23 (4.8125, 24.45) -> (-4.8125, 24.45)
  line L24 (-4.8125, 24.45) -> (-4.8125, 30.45)
  line L25 (-4.8125, 30.45) -> (4.8125, 30.45)
  line L26 (4.8125, 30.45) -> (4.8125, 24.45)
  line L27 (0, 27.95) -> (0, 30.45)
  line L28 (0, 26.95) -> (0, 24.45)
  line L29 (-1.875, 27.95) -> (1.875, 27.95)
  line L30 (1.875, 27.95) -> (1.875, 30.45)
  line L31 (1.875, 30.45) -> (-1.875, 30.45)
  line L32 (-1.875, 30.45) -> (-1.875, 27.95)
  line L33 (-1.875, 27.95) -> (1.875, 30.45) construction
  line L34 (1.875, 27.95) -> (-1.875, 30.45) construction
  line L35 (-1.875, 26.95) -> (1.875, 26.95)
  line L36 (1.875, 26.95) -> (1.875, 24.45)
  line L37 (1.875, 24.45) -> (-1.875, 24.45)
  line L38 (-1.875, 24.45) -> (-1.875, 26.95)
  line L39 (-1.875, 26.95) -> (1.875, 24.45) construction
  line L40 (1.875, 26.95) -> (-1.875, 24.45) construction
  line L41 (6.0355, 41.7) -> (-6.0355, 41.7) projected
  line L42 (-6.0355, 23.2) -> (6.0355, 23.2) projected
  line L43 (6.0355, 15.7) -> (6.0355, 21.95) projected
  line L44 (-6.0355, 15.7) -> (-6.0355, 21.95) projected
  line L45 (6.0355, 36.45) -> (6.0355, 37.7) projected
  line L46 (-6.0355, 15.7) -> (-6.0355, 21.95) projected
  line L47 (-6.0355, 37.7) -> (-6.0355, 41.7) projected
  line L48 (6.0355, 37.7) -> (6.0355, 41.7) projected
  line L49 (6.0355, 15.7) -> (6.0355, 21.95) projected
  line L50 (-6.0355, 21.95) -> (6.0355, 21.95) projected
  line L51 (0, 13.2) -> (0, 24.45)
  line L52 (0, 30.45) -> (0, 33.3612)
  line L53 (-6.0355, 36.45) -> (-6.0355, 37.7) projected
  line L54 (-6.0355, 23.2) -> (-6.0355, 36.45) projected
  line L55 (6.0355, 37.7) -> (6.0355, 41.7) projected
  line L56 (-6.0355, 37.7) -> (-6.0355, 41.7) projected
  line L57 (-6.0355, 37.7) -> (6.0355, 37.7) projected
  line L58 (6.0355, 36.45) -> (-6.0355, 36.45) projected
  line L59 (6.0355, 21.95) -> (6.0355, 23.2) projected
  line L60 (6.0355, 23.2) -> (6.0355, 36.45) projected
  line L61 (13.25, 15.7) -> (13.25, 13.2) projected
  line L62 (-13.25, 13.2) -> (-13.25, 15.7) projected
  line L63 (-13.25, 13.2) -> (13.25, 13.2) projected
  point P0 (0, 0)
  point P1 (0, 27.45)
  point P2 (0, 29.2)
  point P3 (0, 25.7)
  point P4 (-1.875, 26.2)
  point P5 (1.875, 26.2)
  point P6 (1.875, 28.7)
  point P7 (-1.875, 28.7)
  dimension "d95" = 1
  dimension "d96" = 6.125
  dimension "d97" = 2.5
  dimension "d98" = 1.75
  dimension "d99" = 3.75
  dimension "d100" = 3.75
  dimension "d117" = 11.25
  constraints: 54 end point, 12 midpoint, 8 parallel, 4 perpendicular, 3 horizontal, 2 point on line, 2 vertical, 3 other
  measures "d95" distance of L16.start L16.end
  measures "d96" distance of L19.end L18.end
  measures "d97" distance of L18.end L17.end
  measures "d98" distance between parallel lines of L17 L23
  measures "d99" distance of L31.end L30.end
  measures "d100" distance of L36.end L37.end
  measures "d117" distance of L51.start L28.end
extrude "Extrusion11" add sketch "Sketch6" along normal blind 20 from surface at 17.5 contours L35 L38 L17 L20 L19 L32 L29 L16 | L35 L36 L17 L28 | L28 L17 L38 L35 | L16 L29 L30 L19 L18 L17 L36 L35 | L29 L32 L19 L27 | L27 L19 L30 L29 | L28 L23 L38 L17 | L17 L36 L23 L28 | L27 L25 L30 L19 | L19 L32 L25 L27 | L38 L23 L24 L25 L32 L19 L20 L17 | L17 L18 L19 L30 L25 L26 L23 L36
extrude "Extrusion12" cut sketch "Sketch6" against normal blind 6.125 from surface at 37.5 contours L35 L38 L17 L20 L19 L32 L29 L16 | L35 L36 L17 L28 | L28 L17 L38 L35 | L16 L29 L30 L19 L18 L17 L36 L35 | L29 L32 L19 L27 | L27 L19 L30 L29 | L28 L23 L38 L17 | L17 L36 L23 L28 | L27 L25 L30 L19 | L19 L32 L25 L27
ref_plane "Work Plane5" through (-1.875, 31.375, 27.45) normal (0, 0, 1) x (1, 0, 0)
sketch "Sketch9" plane through (-1.875, 31.375, 27.45) normal (0, 0, 1) x (1, 0, 0)
  line L0 (6.6875, 6.125) -> (19.375, -25.3395)
  line L1 (-2.9375, 6.125) -> (-15.625, -25.3395)
  line L2 (3.75, 6.125) -> (3.75, 0) projected
  line L3 (0, 0) -> (3.75, 0) projected
  line L4 (0, 0) -> (0, 6.125) projected
  line L5 (0, 6.125) -> (-2.9375, 6.125) projected
  line L6 (-2.9375, 6.125) -> (-2.9375, -13.875) projected
  line L7 (6.6875, -13.875) -> (-2.9375, -13.875) projected
  line L8 (6.6875, -13.875) -> (6.6875, 6.125) projected
  line L9 (6.6875, 6.125) -> (3.75, 6.125) projected
  line L10 (-3.9625, -45.5375) -> (7.7125, -45.5375) projected
  line L11 (-13.125, -36.375) -> (-3.9625, -45.5375) projected
  line L12 (-13.125, -26.375) -> (-13.125, -36.375) projected
  line L13 (-3.9625, -17.2125) -> (-13.125, -26.375) projected
  line L14 (7.7125, -17.2125) -> (-3.9625, -17.2125) projected
  line L15 (16.875, -26.375) -> (7.7125, -17.2125) projected
  line L16 (16.875, -36.375) -> (16.875, -26.375) projected
  line L17 (7.7125, -45.5375) -> (16.875, -36.375) projected
  line L18 (-4.1605, -48.875) -> (-15.625, -37.4105) projected
  line L19 (7.9105, -48.875) -> (-4.1605, -48.875) projected
  line L20 (19.375, -37.4105) -> (7.9105, -48.875) projected
  line L21 (19.375, -25.3395) -> (19.375, -37.4105) projected
  line L22 (7.9105, -13.875) -> (19.375, -25.3395) projected
  line L23 (-4.1605, -13.875) -> (7.9105, -13.875) projected
  line L24 (-15.625, -25.3395) -> (-4.1605, -13.875) projected
  line L25 (-15.625, -37.4105) -> (-15.625, -25.3395) projected
  point P0 (1.875, -31.375)
  point P1 (6.6875, -13.875)
  point P2 (-15.625, -25.3395)
  point P3 (-2.9375, -13.875)
  constraints: 4 end point
extrude "Extrusion13" add sketch "Sketch9" along normal mid plane 6 contours L0 L22 L23 L8 | L23 L24 L1 L6
sketch "Sketch8" plane through (0, 0, 0) normal (0, 0, 1) x (1, 0, 0)
  line L0 (-24.725, -16.875) -> (-24.725, 16.875) projected
  line L1 (-22.4775, -16.875) -> (-24.725, -16.875) projected
  line L2 (-16.875, -22.4775) -> (-22.4775, -16.875) projected
  line L3 (-16.875, -24.725) -> (-16.875, -22.4775) projected
  line L4 (16.875, -24.725) -> (-16.875, -24.725) projected
  line L5 (16.875, -22.4775) -> (16.875, -24.725) projected
  line L6 (22.4775, -16.875) -> (16.875, -22.4775) projected
  line L7 (24.725, -16.875) -> (22.4775, -16.875) projected
  line L8 (24.725, 16.875) -> (24.725, -16.875) projected
  line L9 (22.4775, 16.875) -> (24.725, 16.875) projected
  line L10 (16.875, 22.4775) -> (22.4775, 16.875) projected
  line L11 (16.875, 24.725) -> (16.875, 22.4775) projected
  line L12 (-16.875, 24.725) -> (16.875, 24.725) projected
  line L13 (-16.875, 22.4775) -> (-16.875, 24.725) projected
  line L14 (-22.4775, 16.875) -> (-16.875, 22.4775) projected
  line L15 (-24.725, 16.875) -> (-22.4775, 16.875) projected
  line L16 (-14.725, 19.725) -> (-19.725, 14.725) projected
  line L17 (14.725, 19.725) -> (-14.725, 19.725) projected
  line L18 (19.725, 14.725) -> (14.725, 19.725) projected
  line L19 (14.725, -19.725) -> (19.725, -14.725) projected
  line L20 (-14.725, -19.725) -> (14.725, -19.725) projected
  line L21 (-19.725, -14.725) -> (-14.725, -19.725) projected
  line L22 (1.875, 37.5) -> (1.875, 31.375) projected
  line L23 (-1.875, 31.375) -> (-1.875, 37.5) projected
  line L24 (1.875, 34.4375) -> (-1.875, 34.4375)
  circle A0 centre (0, 34.4375) radius 1.875
  circle A1 centre (0, 34.4375) radius 4.3125
  line L25 (16.875, 24.725) -> (2.9256, 37.6058)
  line L26 (-16.875, 24.725) -> (-2.9256, 37.6058)
  line L27 (-19.725, 14.725) -> (-19.725, -14.725) projected
  line L28 (19.725, -14.725) -> (19.725, 14.725) projected
  point P0 (0, 0)
  dimension "d112" = 3.75
  dimension "d113" = 8.625
  constraints: 6 end point, 3 midpoint, 2 centre point, 2 point on circle, 2 tangent, 1 coincident
  measures "d112" diameter of A0
  measures "d113" diameter of A1
extrude "Extrusion14" add sketch "Sketch8" along normal blind 2.5 from surface at 7.7 contours L26 A1 L25 L12 | A1
mirror "Mirror2" about plane through (0, 0, 0) normal (0, 1, 0) of "Extrusion11", "Extrusion12", "Extrusion13", "Extrusion14"
sketch "Sketch10" plane through (24.725, 16.875, 7.7) normal (0, 0, -1) x (-1, 0, 0)
  circle A0 centre (24.725, -51.3125) radius 1.875 projected
  line L0 (44.45, -2.15) -> (44.45, -31.6) projected
  line L1 (44.45, -31.6) -> (39.45, -36.6) projected
  line L2 (39.45, -36.6) -> (10, -36.6) projected
  line L3 (10, -36.6) -> (5, -31.6) projected
  line L4 (5, -31.6) -> (5, -2.15) projected
  line L5 (5, -2.15) -> (10, 2.85) projected
  line L6 (10, 2.85) -> (39.45, 2.85) projected
  line L7 (39.45, 2.85) -> (44.45, -2.15) projected
  circle A1 centre (24.725, 17.5625) radius 1.875 projected
  line L8 (41.6, 7.85) -> (27.6506, 20.7308) projected
  arc A2 (27.6506, 20.7308) -> (21.7994, 20.7308) centre (24.725, 17.5625) ccw projected
  line L9 (21.7994, 20.7308) -> (7.85, 7.85) projected
  line L10 (7.85, 7.85) -> (7.85, 5.6025) projected
  line L11 (7.85, 5.6025) -> (2.2475, 0) projected
  line L12 (2.2475, 0) -> (0, 0) projected
  line L13 (0, 0) -> (0, -33.75) projected
  line L14 (0, -33.75) -> (2.2475, -33.75) projected
  line L15 (2.2475, -33.75) -> (7.85, -39.3525) projected
  line L16 (7.85, -39.3525) -> (7.85, -41.6) projected
  line L17 (21.7994, -54.4808) -> (7.85, -41.6) projected
  arc A3 (21.7994, -54.4808) -> (27.6506, -54.4808) centre (24.725, -51.3125) ccw projected
  line L18 (41.6, -41.6) -> (27.6506, -54.4808) projected
  line L19 (41.6, -41.6) -> (41.6, -39.3525) projected
  line L20 (41.6, -39.3525) -> (47.2025, -33.75) projected
  line L21 (47.2025, -33.75) -> (49.45, -33.75) projected
  line L22 (49.45, -33.75) -> (49.45, 0) projected
  line L23 (49.45, 0) -> (47.2025, 0) projected
  line L24 (47.2025, 0) -> (41.6, 5.6025) projected
  line L25 (41.6, 5.6025) -> (41.6, 7.85) projected
  line L26 (49.45, -31.6) -> (44.45, -31.6)
  line L27 (44.45, -31.6) -> (44.45, -2.15)
  line L28 (44.45, -2.15) -> (49.45, -2.15)
  line L29 (49.45, -2.15) -> (49.45, -31.6)
  line L30 (5, -31.6) -> (0, -31.6)
  line L31 (0, -31.6) -> (0, -2.15)
  line L32 (0, -2.15) -> (5, -2.15)
  line L33 (5, -2.15) -> (5, -31.6)
  point P0 (24.725, -16.875)
  point P1 (5, -2.15)
  point P2 (0, -31.6)
  point P3 (49.45, -2.15)
  dimension "d125" = 29.45
  constraints: 16 end point, 4 parallel, 2 horizontal, 2 perpendicular, 2 point on line
  measures "d125" distance of L30.end L31.end
extrude "Extrusion16" cut sketch "Sketch10" against normal up to surface (2.5 mm away) contours L28 L22 L26 L0 | L4 L30 L13 L32
sketch "Sketch11" plane through (0, 0, 0) normal (1, 0, 0) x (0, 1, 0)
  line L0 (15.6625, 13.2) -> (15.6625, 8.2) projected
  line L1 (15.6625, 8.2) -> (12.6625, 8.2) projected
  line L2 (12.6625, 8.2) -> (12.6625, 13.2) projected
  line L3 (15.6625, 13.2) -> (12.6625, 13.2) projected
  line L4 (-12.6625, 8.2) -> (-12.6625, 13.2) projected
  line L5 (-12.6625, 8.2) -> (-15.6625, 8.2) projected
  line L6 (-15.6625, 8.2) -> (-15.6625, 13.2) projected
  line L7 (-12.6625, 13.2) -> (-15.6625, 13.2) projected
  line L8 (12.6625, 13.2) -> (12.7875, 13.2)
  line L9 (12.7875, 13.2) -> (12.6625, 8.2)
  line L10 (-12.6625, 13.2) -> (-12.7875, 13.2)
  line L11 (-12.7875, 13.2) -> (-12.6625, 8.2)
  point P0 (0, 0)
  dimension "d128" = 0.125
  dimension "d129" = 0.125
  constraints: 8 end point, 2 point on line
  measures "d128" distance of L2.end L8.end
  measures "d129" distance of L4.end L10.end
extrude "Extrusion17" cut sketch "Sketch11" along normal up to surface (20 mm away) from surface at -10 contours L9 L2 L3 | L11 L7 L4
chamfer "Chamfer4" distance 5 angle 45 4 edges at (10, 14.225, 13.2) (10, -14.225, 13.2) (-10, 14.225, 13.2) (-10, -14.225, 13.2)
equation "\"d27\" = d26"
equation "\"d15\" = d14"
equation "\"d37\" = d36"
equation "\"d38\" = d36"
equation "\"d39\" = d38"
equation "\"d40\" = d36"
equation "\"d41\" = d40"
equation "\"d42\" = d36"
equation "\"d43\" = d42"
equation "\"d60\" = d59"
equation "\"d61\" = d59"
equation "\"d62\" = d61"
equation "\"d63\" = d59"
equation "\"d64\" = d63"
equation "\"d65\" = d59"
equation "\"d66\" = d65"
body "Solid1"
